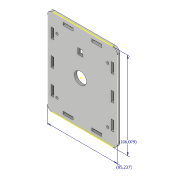
# Autodesk Inventor part: tapa2
Saved by Autodesk Inventor 2019 (Build 230136000, 136)
## iProperties
Created: 2018-09-20
Part Number: tapa2
Material: Genérico
Document SubType Name: Modeling
Designer: lmacia
Density: 1 g/cm^3
Appearance: Valor por defecto
Author: lmacia
Autodesk Inventor part; units mm, degrees
ref_plane "YZ Plane" through (0, 0, 0) normal (1, 0, 0) x (0, 1, 0)
ref_plane "XZ Plane" through (0, 0, 0) normal (0, 1, 0) x (-1, 0, 0)
ref_plane "XY Plane" through (0, 0, 0) normal (0, 0, 1) x (1, 0, 0)
sketch "Boceto1" plane through (0, 0, 0) normal (0, 0, 1) x (-1, 0, 0)
  line L0 (-40.5654, -5.9984) -> (-40.5654, 6.2017)
  line L1 (-40.5654, 6.2017) -> (-40.4637, 6.2017)
  line L2 (-40.4637, 6.2017) -> (-37.4137, 6.2017)
  line L3 (-37.4137, 6.2017) -> (-37.312, 6.2017)
  line L4 (-37.312, 6.2017) -> (-37.312, -5.9984)
  line L5 (-37.312, -5.9984) -> (-37.4137, -5.9984)
  line L6 (-37.4137, -5.9984) -> (-40.4637, -5.9984)
  line L7 (-40.4637, -5.9984) -> (-40.5654, -5.9984)
  line L8 (35.787, -5.9984) -> (35.6854, -5.9984)
  line L9 (35.6854, -5.9984) -> (32.6353, -5.9984)
  line L10 (32.6353, -5.9984) -> (32.5337, -5.9984)
  line L11 (32.5337, -5.9984) -> (32.5337, 6.2017)
  line L12 (32.5337, 6.2017) -> (32.6353, 6.2017)
  line L13 (32.6353, 6.2017) -> (35.6854, 6.2017)
  line L14 (35.6854, 6.2017) -> (35.787, 6.2017)
  line L15 (35.787, 6.2017) -> (35.787, -5.9984)
  line L16 (35.6854, 36.4987) -> (35.787, 36.4987)
  line L17 (35.787, 36.4987) -> (35.787, 24.2986)
  line L18 (35.787, 24.2986) -> (35.6854, 24.2986)
  line L19 (35.6854, 24.2986) -> (32.6353, 24.2986)
  line L20 (32.6353, 24.2986) -> (32.5337, 24.2986)
  line L21 (32.5337, 24.2986) -> (32.5337, 36.4987)
  line L22 (32.5337, 36.4987) -> (32.6353, 36.4987)
  line L23 (32.6353, 36.4987) -> (35.6854, 36.4987)
  line L24 (-26.0015, -48.4955) -> (-26.0015, -48.3938)
  line L25 (-26.0015, -48.3938) -> (-26.0015, -45.3438)
  line L26 (-26.0015, -45.3438) -> (-26.0015, -45.2421)
  line L27 (-26.0015, -45.2421) -> (-13.8014, -45.2421)
  line L28 (-13.8014, -45.2421) -> (-13.8014, -45.3438)
  line L29 (-13.8014, -45.3438) -> (-13.8014, -48.3938)
  line L30 (-13.8014, -48.3938) -> (-13.8014, -48.4955)
  line L31 (-13.8014, -48.4955) -> (-26.0015, -48.4955)
  line L32 (9.023, 45.4455) -> (9.023, 45.5471)
  line L33 (9.023, 45.5471) -> (9.023, 48.5971)
  line L34 (9.023, 48.5971) -> (9.023, 48.6988)
  line L35 (9.023, 48.6988) -> (21.2231, 48.6988)
  line L36 (21.2231, 48.6988) -> (21.2231, 48.5971)
  line L37 (21.2231, 48.5971) -> (21.2231, 45.5471)
  line L38 (21.2231, 45.5471) -> (21.2231, 45.4455)
  line L39 (21.2231, 45.4455) -> (9.023, 45.4455)
  line L40 (-26.0015, 45.4455) -> (-26.0015, 45.5471)
  line L41 (-26.0015, 45.5471) -> (-26.0015, 48.5971)
  line L42 (-26.0015, 48.5971) -> (-26.0015, 48.6988)
  line L43 (-26.0015, 48.6988) -> (-13.8014, 48.6988)
  line L44 (-13.8014, 48.6988) -> (-13.8014, 48.5971)
  line L45 (-13.8014, 48.5971) -> (-13.8014, 45.5471)
  line L46 (-13.8014, 45.5471) -> (-13.8014, 45.4455)
  line L47 (-13.8014, 45.4455) -> (-26.0015, 45.4455)
  line L48 (32.6353, -24.0952) -> (35.6854, -24.0952)
  line L49 (35.6854, -24.0952) -> (35.787, -24.0952)
  line L50 (35.787, -24.0952) -> (35.787, -36.2954)
  line L51 (35.787, -36.2954) -> (35.6854, -36.2954)
  line L52 (35.6854, -36.2954) -> (32.6353, -36.2954)
  line L53 (32.6353, -36.2954) -> (32.5337, -36.2954)
  line L54 (32.5337, -36.2954) -> (32.5337, -24.0952)
  line L55 (32.5337, -24.0952) -> (32.6353, -24.0952)
  line L56 (9.023, -48.4955) -> (9.023, -48.3938)
  line L57 (9.023, -48.3938) -> (9.023, -45.3438)
  line L58 (9.023, -45.3438) -> (9.023, -45.2421)
  line L59 (9.023, -45.2421) -> (21.2231, -45.2421)
  line L60 (21.2231, -45.2421) -> (21.2231, -45.3438)
  line L61 (21.2231, -45.3438) -> (21.2231, -48.3938)
  line L62 (21.2231, -48.3938) -> (21.2231, -48.4955)
  line L63 (21.2231, -48.4955) -> (9.023, -48.4955)
  line L64 (-37.4137, -36.2954) -> (-40.4637, -36.2954)
  line L65 (-40.4637, -36.2954) -> (-40.5654, -36.2954)
  line L66 (-40.5654, -36.2954) -> (-40.5654, -24.0952)
  line L67 (-40.5654, -24.0952) -> (-40.4637, -24.0952)
  line L68 (-40.4637, -24.0952) -> (-37.4137, -24.0952)
  line L69 (-37.4137, -24.0952) -> (-37.312, -24.0952)
  line L70 (-37.312, -24.0952) -> (-37.312, -36.2954)
  line L71 (-37.312, -36.2954) -> (-37.4137, -36.2954)
  line L72 (-37.312, 36.4987) -> (-37.312, 24.2986)
  line L73 (-37.312, 24.2986) -> (-37.4137, 24.2986)
  line L74 (-37.4137, 24.2986) -> (-40.4637, 24.2986)
  line L75 (-40.4637, 24.2986) -> (-40.5654, 24.2986)
  line L76 (-40.5654, 24.2986) -> (-40.5654, 36.4987)
  line L77 (-40.5654, 36.4987) -> (-40.4637, 36.4987)
  line L78 (-40.4637, 36.4987) -> (-37.4137, 36.4987)
  line L79 (-37.4137, 36.4987) -> (-37.312, 36.4987)
  line L80 (-3.05, -23.6886) -> (3.05, -23.6886)
  line L81 (3.05, -23.6886) -> (3.05, -30.8053)
  line L82 (3.05, -30.8053) -> (-3.05, -30.8053)
  line L83 (-3.05, -30.8053) -> (-3.05, -23.6886)
  circle A0 centre (-33.347, 34.9737) radius 1.4233
  circle A1 centre (28.5686, 34.9737) radius 1.4233
  circle A2 centre (0, 0) radius 7.3709
  circle A3 centre (-33.347, -32.6353) radius 1.4233
  circle A4 centre (28.5686, -32.6353) radius 1.4233
  line L84 (21.2231, 48.6988) -> (9.023, 48.6988)
  line L85 (9.023, 48.6988) -> (9.023, 45.4455)
  line L86 (9.023, 45.4455) -> (21.2231, 45.4455)
  line L87 (21.2231, 45.4455) -> (21.2231, 48.6988)
  line L88 (35.787, 36.4987) -> (32.5337, 36.4987)
  line L89 (32.5337, 36.4987) -> (32.5337, 24.2986)
  line L90 (32.5337, 24.2986) -> (35.787, 24.2986)
  line L91 (35.787, 24.2986) -> (35.787, 36.4987)
  line L92 (35.787, 6.2017) -> (32.5337, 6.2017)
  line L93 (32.5337, 6.2017) -> (32.5337, -5.9984)
  line L94 (32.5337, -5.9984) -> (35.787, -5.9984)
  line L95 (35.787, -5.9984) -> (35.787, 6.2017)
  line L96 (35.787, -24.0952) -> (32.5337, -24.0952)
  line L97 (32.5337, -24.0952) -> (32.5337, -36.2954)
  line L98 (32.5337, -36.2954) -> (35.787, -36.2954)
  line L99 (35.787, -36.2954) -> (35.787, -24.0952)
  line L100 (21.2231, -45.2421) -> (9.023, -45.2421)
  line L101 (9.023, -45.2421) -> (9.023, -48.4955)
  line L102 (9.023, -48.4955) -> (21.2231, -48.4955)
  line L103 (21.2231, -48.4955) -> (21.2231, -45.2421)
  line L104 (-13.8014, -45.2421) -> (-26.0015, -45.2421)
  line L105 (-26.0015, -45.2421) -> (-26.0015, -48.4955)
  line L106 (-26.0015, -48.4955) -> (-13.8014, -48.4955)
  line L107 (-13.8014, -48.4955) -> (-13.8014, -45.2421)
  line L108 (-37.312, -36.2954) -> (-40.5654, -36.2954)
  line L109 (-40.5654, -36.2954) -> (-40.5654, -24.0952)
  line L110 (-40.5654, -24.0952) -> (-37.312, -24.0952)
  line L111 (-37.312, -24.0952) -> (-37.312, -36.2954)
  line L112 (-37.312, -5.9984) -> (-40.5654, -5.9984)
  line L113 (-40.5654, -5.9984) -> (-40.5654, 6.2017)
  line L114 (-40.5654, 6.2017) -> (-37.312, 6.2017)
  line L115 (-37.312, 6.2017) -> (-37.312, -5.9984)
  line L116 (-37.312, 24.2986) -> (-40.5654, 24.2986)
  line L117 (-40.5654, 24.2986) -> (-40.5654, 36.4987)
  line L118 (-40.5654, 36.4987) -> (-37.312, 36.4987)
  line L119 (-37.312, 36.4987) -> (-37.312, 24.2986)
  line L120 (-26.0015, 48.6988) -> (-13.8014, 48.6988)
  line L121 (-13.8014, 48.6988) -> (-13.8014, 45.4455)
  line L122 (-13.8014, 45.4455) -> (-26.0015, 45.4455)
  line L123 (-26.0015, 45.4455) -> (-26.0015, 48.6988)
  line L124 (3.05, -23.6886) -> (-3.05, -23.6886)
  line L125 (-3.05, -23.6886) -> (-3.05, -30.8053)
  line L126 (-3.05, -30.8053) -> (3.05, -30.8053)
  line L127 (3.05, -30.8053) -> (3.05, -23.6886)
  arc A5 (40.2295, 47.3577) -> (34.4459, 53.1413) centre (34.4459, 47.3577) ccw
  line L128 (34.4459, 53.1413) -> (-39.2245, 53.1413)
  arc A6 (-39.2245, 53.1413) -> (-45.0078, 47.3579) centre (-39.2245, 47.3579) ccw
  line L129 (-45.0078, 47.3579) -> (-45.0078, -47.1423)
  arc A7 (-45.0078, -47.1423) -> (-39.2123, -52.9379) centre (-39.2123, -47.1423) ccw
  line L130 (-39.2123, -52.9379) -> (34.4339, -52.9379)
  arc A8 (34.4339, -52.9379) -> (40.2295, -47.1423) centre (34.4339, -47.1423) ccw
  line L131 (40.2295, -47.1423) -> (40.2295, 47.3577)
  constraints: 264 end point, 22 parallel, 13 horizontal, 11 perpendicular, 9 centre point, 8 point on circle, 8 tangent, 2 vertical
extrude "Extrusión1" add sketch "Boceto1" along normal blind 3
sketch "Boceto2" plane through (0, 0, 3) normal (0, 0, 1) x (1, 0, 0)
  line L0 (-34.4459, -53.1413) -> (39.2245, -53.1413) projected
  line L1 (39.2123, 52.9379) -> (-34.4339, 52.9379) projected
  line L2 (-40.2295, 47.1423) -> (-40.2295, -47.3577) projected
  line L3 (45.0078, -47.3579) -> (45.0078, 47.1423) projected
  point P0 (0, 0)
  dimension "d5" = 106.0792
  dimension "d6" = 85.2373
  measures "d5" distance between parallel lines of L0 L1
  measures "d6" distance between parallel lines of L2 L3
